Autodesk Inventor part; units mm, degrees
(part 2 of 2)
sketch "Sketch120" plane through (0, 0, 52) normal (0, 0, -1) x (-1, 0, 0)
  line L0 (-5.5, 48.7965) -> (-5.5, 49.7965) projected
  line L1 (-5.5, 47.9965) -> (-5.5, 48.7965) projected
  line L2 (-5.5, 47.9965) -> (-5.5, 45.9965) projected
  line L3 (-5.5, 45.9965) -> (-5.5, 19.7965) projected
  line L4 (-5.5, 19.7965) -> (-5.5, 45.9965) projected
  line L5 (-5.5, 45.9965) -> (-5.5, 47.9965) projected
  line L6 (-5.5, 48.7965) -> (-5.5, 47.9965) projected
  line L7 (-5.5, 49.7965) -> (-5.5, 48.7965) projected
  line L8 (-5.5, -48.7965) -> (-5.5, -49.7965) projected
  line L9 (-5.5, -47.9965) -> (-5.5, -48.7965) projected
  line L10 (-5.5, -47.9965) -> (-5.5, -45.9965) projected
  line L11 (-5.5, -45.9965) -> (-5.5, -19.7965) projected
  line L12 (-5.5, -19.7965) -> (-5.5, -45.9965) projected
  line L13 (-5.5, -45.9965) -> (-5.5, -47.9965) projected
  line L14 (-5.5, -48.7965) -> (-5.5, -47.9965) projected
  line L15 (-5.5, -49.7965) -> (-5.5, -48.7965) projected
  line L16 (-6, 5.3855) -> (-6, 46.7965) projected
  line L17 (-6, -46.7965) -> (-6, -5.3855) projected
  line L18 (-6, 46.7965) -> (-3.5, 46.7965)
  line L19 (-3.5, 46.7965) -> (-3.5, 17.7965)
  line L20 (-3.5, 17.7965) -> (-6, 17.7965)
  line L21 (-6, 17.7965) -> (-6, 46.7965)
  line L22 (-6, -46.7965) -> (-3.5, -46.7965)
  line L23 (-3.5, -46.7965) -> (-3.5, -17.7965)
  line L24 (-3.5, -17.7965) -> (-6, -17.7965)
  line L25 (-6, -17.7965) -> (-6, -46.7965)
  point P0 (0, 0)
  dimension "d491" = 2
  dimension "d492" = 2
  dimension "d493" = 2
  constraints: 16 end point, 4 parallel, 2 horizontal, 2 perpendicular, 1 vertical alignment
  measures "d491" distance between parallel lines of L19 L3
  measures "d492" distance from line of L20 L3.end
  measures "d493" distance from line of L24 L11.end
extrude "Extrusion103" add sketch "Sketch120" along normal blind 2
sketch "Sketch123" plane through (9, -49.7965, 50) normal (1, 0, 0) x (0, 0, -1)
  line L0 (-2, 99.5929) -> (-5, 99.5929)
  line L1 (-5, 99.5929) -> (-5, 69.5929)
  line L2 (-5, 69.5929) -> (-2, 69.5929)
  line L3 (-2, 69.5929) -> (-2, 99.5929)
  line L4 (-3, 69.5929) -> (-32, 69.5929) projected
  line L5 (-3, 98.5929) -> (-3, 97.7929) projected
  line L6 (-3, 69.5929) -> (-35, 69.5929) projected
  line L7 (-19, 69.5929) -> (-19, 30)
  line L8 (-35, 30) -> (-3, 30) projected
  line L9 (0, 49.7965) -> (-70, 49.7965) projected
  line L10 (-2, 0) -> (-5, 0)
  line L11 (-5, 0) -> (-5, 30)
  line L12 (-5, 30) -> (-2, 30)
  line L13 (-2, 30) -> (-2, 0)
  line L14 (-36, 99.5929) -> (-33, 99.5929)
  line L15 (-33, 99.5929) -> (-33, 69.5929)
  line L16 (-33, 69.5929) -> (-36, 69.5929)
  line L17 (-36, 69.5929) -> (-36, 99.5929)
  line L18 (-33, 0) -> (-33, 30)
  line L19 (-36, 30) -> (-36, 0)
  line L20 (-33, 30) -> (-36, 30)
  line L21 (-36, 0) -> (-33, 0)
  point P0 (50, 49.7965)
  dimension "d494" = 2
  constraints: 34 end point, 12 symmetric about line, 2 midpoint, 2 parallel, 1 horizontal, 1 perpendicular, 1 point on line
  measures "d494" distance between parallel lines of L1 L5
extrude "Extrusion105" add sketch "Sketch123" against normal blind 1
sketch "Sketch125" plane through (5.5, -49.7965, 50) normal (1, 0, 0) x (0, 0, -1)
  line L0 (-36, 99.5929) -> (-2, 99.5929) projected
  line L1 (-35, 98.5929) -> (-36, 99.5929) projected
  line L2 (-35, 97.7929) -> (-35, 98.5929) projected
  line L3 (-35, 97.7929) -> (-35.6, 97.7929) projected
  line L4 (-35.6, 97.7929) -> (-35.6, 95.7929) projected
  line L5 (-35.6, 95.7929) -> (-35, 69.5929) projected
  line L6 (-3, 69.5929) -> (-35, 69.5929) projected
  line L7 (-3, 69.5929) -> (-2.4, 95.7929) projected
  line L8 (-2.4, 95.7929) -> (-2.4, 97.7929) projected
  line L9 (-2.4, 97.7929) -> (-3, 97.7929) projected
  line L10 (-3, 98.5929) -> (-3, 97.7929) projected
  line L11 (-2, 99.5929) -> (-3, 98.5929) projected
  line L12 (-2, 0) -> (-36, 0) projected
  line L13 (-3, 1) -> (-2, 0) projected
  line L14 (-3, 1.8) -> (-3, 1) projected
  line L15 (-3, 1.8) -> (-2.4, 1.8) projected
  line L16 (-2.4, 1.8) -> (-2.4, 3.8) projected
  line L17 (-2.4, 3.8) -> (-3, 30) projected
  line L18 (-35, 30) -> (-3, 30) projected
  line L19 (-35, 30) -> (-35.6, 3.8) projected
  line L20 (-35.6, 3.8) -> (-35.6, 1.8) projected
  line L21 (-35.6, 1.8) -> (-35, 1.8) projected
  line L22 (-35, 1) -> (-35, 1.8) projected
  line L23 (-36, 0) -> (-35, 1) projected
  point P0 (50, 49.7965)
extrude "Extrusion106" cut sketch "Sketch125" against normal blind 1
sketch "Sketch126" plane through (0, 0, 52) normal (0, 0, -1) x (-1, 0, 0)
  line L0 (21, 25.6491) -> (10, 19.2983)
  line L1 (10, 19.2983) -> (-1, 25.6491)
  line L2 (-1, 25.6491) -> (-1, 38.3509)
  line L3 (-1, 38.3509) -> (10, 44.7017)
  line L4 (10, 44.7017) -> (21, 38.3509)
  line L5 (21, 38.3509) -> (21, 25.6491)
  line L6 (0, 0) -> (77.78, 0) construction
  line L7 (21, -25.6491) -> (10, -19.2983)
  line L8 (10, -19.2983) -> (-1, -25.6491)
  line L9 (-1, -25.6491) -> (-1, -38.3509)
  line L10 (-1, -38.3509) -> (10, -44.7017)
  line L11 (10, -44.7017) -> (21, -38.3509)
  line L12 (21, -38.3509) -> (21, -25.6491)
  point P0 (10, 32)
  dimension "d499" = 32
  dimension "d500" = 22
  dimension "d501" = 10
  constraints: 26 end point, 6 symmetric about line, 1 horizontal, 1 vertical, 13 other
  measures "d499" vertical distance of L6.start point (10, 32)
  measures "d500" distance between parallel lines of L2 L5
  measures "d501" horizontal distance of L6.start point (10, 32)
extrude "Extrusion107" cut sketch "Sketch126" against normal through all
sketch "Sketch128" plane through (4.5, -49.7965, 50) normal (1, 0, 0) x (0, 0, -1)
  line L0 (-36, 99.5929) -> (-2, 99.5929) construction
  line L1 (-35, 98.5929) -> (-36, 99.5929) projected
  line L2 (-35, 97.7929) -> (-35, 98.5929) projected
  line L3 (-35.6, 97.7929) -> (-35, 97.7929) projected
  line L4 (-35.6, 95.7929) -> (-35.6, 97.7929) projected
  line L5 (-35, 69.5929) -> (-35.6, 95.7929) projected
  line L6 (-3, 69.5929) -> (-35, 69.5929) projected
  line L7 (-2.4, 95.7929) -> (-3, 69.5929) projected
  line L8 (-2.4, 97.7929) -> (-2.4, 95.7929) projected
  line L9 (-3, 97.7929) -> (-2.4, 97.7929) projected
  line L10 (-3, 98.5929) -> (-3, 97.7929) projected
  line L11 (-2, 99.5929) -> (-3, 98.5929) projected
  line L12 (-2.4, 97.7929) -> (-2.4, 99.1929)
  line L13 (-2.4, 99.1929) -> (-3, 98.5929)
  line L14 (-3, 98.5929) -> (-3, 97.7929)
  line L15 (-2.4, 97.7929) -> (-3, 97.7929)
  line L16 (-35.6, 97.7929) -> (-35.6, 99.1929)
  line L17 (-35.6, 99.1929) -> (-35, 98.5929)
  line L18 (-35, 97.7929) -> (-35, 98.5929)
  line L19 (-35, 97.7929) -> (-35.6, 97.7929)
  point P0 (50, 49.7965)
  constraints: 16 end point, 5 collinear, 2 point on line, 1 parallel, 1 perpendicular, 1 vertical
extrude "Extrusion108" cut sketch "Sketch128" along normal blind 3.5
sketch "Sketch129" plane through (4.5, -49.7965, 50) normal (1, 0, 0) x (0, 0, -1)
  line L0 (-36, 99.5929) -> (-2, 99.5929) projected
  line L1 (-35.6, 99.1929) -> (-36, 99.5929) projected
  line L2 (-35.6, 99.1929) -> (-35.6, 95.7929) projected
  line L3 (-35, 69.5929) -> (-35.6, 95.7929) projected
  line L4 (-3, 69.5929) -> (-35, 69.5929) construction
  line L5 (-2.4, 95.7929) -> (-3, 69.5929) projected
  line L6 (-2.4, 99.1929) -> (-2.4, 95.7929) projected
  line L7 (-2, 99.5929) -> (-2.4, 99.1929) projected
  line L8 (-35, 69.5929) -> (-35, 99.5929)
  line L9 (-35, 99.5929) -> (-3, 99.5929)
  line L10 (-3, 99.5929) -> (-3, 69.5929)
  line L11 (-35, 99.5929) -> (-34, 99.5929)
  line L12 (-34, 99.5929) -> (-34, 97.5929)
  line L13 (-34, 97.5929) -> (-35, 97.5929)
  line L14 (-35, 97.5929) -> (-35, 99.5929)
  line L15 (-35, 99.5929) -> (-36, 99.5929)
  line L16 (-35, 97.5929) -> (-36, 97.5929)
  line L17 (-36, 97.5929) -> (-36, 99.5929)
  point P0 (50, 49.7965)
  dimension "d506" = 1
  dimension "d507" = 28
  dimension "d508" = 2
  constraints: 20 end point, 4 parallel, 4 perpendicular, 3 point on line, 2 horizontal
  measures "d506" distance of L12.end L13.end
  measures "d507" distance between parallel lines of L4 L13
  measures "d508" distance of L11.end L12.end
extrude "Extrusion109" add sketch "Sketch129" along normal blind 3.5 contours L0 L8 L16 L2 L1 | L1 L2 L16 L17 | L0 L12 L13 L8
mirror "Mirror1" about plane through (0, 0, 0) normal (0, 1, 0) of "Extrusion108", "Extrusion109"
chamfer "Chamfer4" distance 1 angle 45 2 edges at (6.25, -49.7965, 84) (6.25, 49.7965, 84)
sketch "Sketch131" plane through (0, 0, 82) normal (0, 0, -1) x (-1, 0, 0)
  circle A0 centre (-30, 0) radius 16.5 projected
  line L0 (-27.0179, 46.7965) -> (-9, 46.7965) projected
  line L1 (-54.0359, 0) -> (-27.0179, 46.7965) projected
  line L2 (-27.0179, -46.7965) -> (-54.0359, 0) projected
  line L3 (-9, -46.7965) -> (-27.0179, -46.7965) projected
  line L4 (-9, -19.7965) -> (-9, -46.7965) projected
  line L5 (-9, 19.7965) -> (-9, -19.7965) projected
  line L6 (-9, 46.7965) -> (-9, 19.7965) projected
  point P0 (0, 0)
extrude "Extrusion111" add sketch "Sketch131" along normal blind 2
sketch "Sketch132" plane through (0, 0, 52) normal (0, 0, -1) x (-1, 0, 0)
  line L0 (21, 38.3509) -> (21, 25.6491) projected
  line L1 (21, 25.6491) -> (10, 19.2983) projected
  line L2 (10, 19.2983) -> (-1, 25.6491) projected
  line L3 (-1, 25.6491) -> (-1, 38.3509) projected
  line L4 (-1, 38.3509) -> (10, 44.7017) projected
  line L5 (10, 44.7017) -> (21, 38.3509) projected
  line L6 (21, -25.6491) -> (21, -38.3509) projected
  line L7 (21, -38.3509) -> (10, -44.7017) projected
  line L8 (10, -44.7017) -> (-1, -38.3509) projected
  line L9 (-1, -38.3509) -> (-1, -25.6491) projected
  line L10 (-1, -25.6491) -> (10, -19.2983) projected
  line L11 (10, -19.2983) -> (21, -25.6491) projected
  arc A0 (38.8444, 24.1666) -> (21.1556, 24.1666) centre (30, 19.5) ccw projected
  line L12 (45, 12.5) -> (38.8444, 24.1666) projected
  line L13 (45, -12.5) -> (45, 12.5) projected
  line L14 (38.5, -12.5) -> (45, -12.5) projected
  line L15 (38.5, -19.5) -> (38.5, -12.5) projected
  line L16 (21.5, -19.5) -> (38.5, -19.5) projected
  line L17 (21.5, -12.5) -> (21.5, -19.5) projected
  line L18 (15, -12.5) -> (21.5, -12.5) projected
  line L19 (15, 12.5) -> (15, -12.5) projected
  line L20 (21.1556, 24.1666) -> (15, 12.5) projected
  line L21 (-3.5, 46.7965) -> (-3.5, 17.7965) projected
  line L22 (-3.5, 17.7965) -> (-6, 17.7965) projected
  line L23 (-6, 17.7965) -> (-6, 5.3855) projected
  arc A1 (-6, -5.3855) -> (-6, 5.3855) centre (0, 0) ccw projected
  line L24 (-6, -17.7965) -> (-6, -5.3855) projected
  line L25 (-6, -17.7965) -> (-3.5, -17.7965) projected
  line L26 (-3.5, -17.7965) -> (-3.5, -46.7965) projected
  line L27 (-3.5, -46.7965) -> (27.0179, -46.7965) projected
  line L28 (27.0179, -46.7965) -> (54.0359, 0) projected
  line L29 (27.0179, 46.7965) -> (54.0359, 0) projected
  line L30 (27.0179, 46.7965) -> (-3.5, 46.7965) projected
extrude "Extrusion112" add sketch "Sketch132" along normal blind 2
sketch "Sketch134" plane through (0, 0, 50) normal (0, 0, -1) x (-1, 0, 0)
  line L0 (21, 38.3509) -> (21, 25.6491) projected
  line L1 (21, 25.6491) -> (10, 19.2983) projected
  line L2 (21, 25.6491) -> (10, 19.2983) projected
  line L3 (10, 19.2983) -> (-1, 25.6491) projected
  line L4 (-1, 25.6491) -> (-1, 38.3509) projected
  line L5 (-1, 38.3509) -> (10, 44.7017) projected
  line L6 (10, 44.7017) -> (21, 38.3509) projected
  line L7 (21, 38.3509) -> (21, 25.6491) projected
  line L8 (21, -38.3509) -> (10, -44.7017) projected
  line L9 (10, -44.7017) -> (-1, -38.3509) projected
  line L10 (-1, -38.3509) -> (-1, -25.6491) projected
  line L11 (-1, -25.6491) -> (10, -19.2983) projected
  line L12 (10, -19.2983) -> (21, -25.6491) projected
  line L13 (21, -25.6491) -> (21, -38.3509) projected
  line L14 (38.8444, 24.1666) -> (45, 12.5) projected
  line L15 (45, 12.5) -> (45, -12.5) projected
  line L16 (45, -12.5) -> (38.5, -12.5) projected
  line L17 (38.5, -12.5) -> (38.5, -19.5) projected
  line L18 (38.5, -19.5) -> (21.5, -19.5) projected
  line L19 (21.5, -19.5) -> (21.5, -12.5) projected
  line L20 (21.5, -12.5) -> (15, -12.5) projected
  line L21 (15, -12.5) -> (15, 12.5) projected
  line L22 (15, 12.5) -> (21.1556, 24.1666) projected
  arc A0 (38.8444, 24.1666) -> (21.1556, 24.1666) centre (30, 19.5) ccw projected
  circle A1 centre (0, 0) radius 8.0625 projected
  line L23 (28.75, -49.7965) -> (57.5, 0) projected
  line L24 (28.75, 49.7965) -> (57.5, 0) projected
  line L25 (28.75, 49.7965) -> (-9, 49.7965) projected
  line L26 (-9, 49.7965) -> (-9, -49.7965) projected
  line L27 (-9, -49.7965) -> (28.75, -49.7965) projected
extrude "Extrusion113" add sketch "Sketch134" against normal blind 70 contours L0 L1 L3 L4 L5 L6 | L8 L9 L10 L11 L12 L13
sketch "Sketch135" plane through (0, 0, 50) normal (0, 0, -1) x (-1, 0, 0)
  circle A0 centre (0, 0) radius 42.5 construction
  circle A1 centre (26.2333, -33.4374) radius 3.5 construction
  circle A2 centre (15.841, -39.4374) radius 3.5 construction
  circle A3 centre (-17.8508, -38.5694) radius 3.5 construction
  circle A4 centre (-30.1381, -29.9658) radius 3.5 construction
  line L0 (26.2333, -33.4374) -> (15.841, -39.4374)
  line L1 (-17.8508, -38.5694) -> (-30.1381, -29.9658)
  line L2 (0, 0) -> (21.0372, -36.4374) construction
  line L3 (21.0372, -36.4374) -> (-23.9944, -34.2676) construction
  line L4 (0, 0) -> (-23.9944, -34.2676) construction
  line L5 (0, 0) -> (16.8866, 0) construction
  circle A5 centre (26.2333, 33.4374) radius 3.5 construction
  circle A6 centre (15.841, 39.4374) radius 3.5 construction
  circle A7 centre (-17.8508, 38.5694) radius 3.5 construction
  circle A8 centre (-30.1381, 29.9658) radius 3.5 construction
  circle A9 centre (0, 0) radius 39 construction
  circle A10 centre (0, 0) radius 46 construction
  arc A11 (30.8761, -34.0979) -> (26.1775, -28.9091) centre (28.5268, -31.5035) ccw
  arc A12 (11.9473, -37.125) -> (14.0917, -43.7884) centre (13.0195, -40.4567) ccw
  arc A13 (14.0917, -43.7884) -> (30.8761, -34.0979) centre (0, 0) ccw
  arc A14 (11.9473, -37.125) -> (26.1775, -28.9091) centre (0, 0) ccw
  line L6 (23, -39.8372) -> (19.5, -33.775)
  arc A15 (-16.3278, -43.0047) -> (-13.8431, -36.4605) centre (-15.0855, -39.7326) ccw
  arc A16 (-29.527, -25.4785) -> (-34.8268, -30.0516) centre (-32.1769, -27.765) ccw
  arc A17 (-29.527, -25.4785) -> (-13.8431, -36.4605) centre (0, 0) ccw
  arc A18 (-34.8268, -30.0516) -> (-16.3278, -43.0047) centre (0, 0) ccw
  circle A19 centre (26.2333, 33.4374) radius 3.5 construction
  line L7 (26.2333, 33.4374) -> (15.841, 39.4374)
  circle A20 centre (15.841, 39.4374) radius 3.5 construction
  line L8 (21.0372, 36.4374) -> (-23.9944, 34.2676) construction
  circle A21 centre (-17.8508, 38.5694) radius 3.5 construction
  circle A22 centre (-30.1381, 29.9658) radius 3.5 construction
  line L9 (-17.8508, 38.5694) -> (-30.1381, 29.9658)
  arc A23 (26.1775, 28.9091) -> (30.8761, 34.0979) centre (28.5268, 31.5035) ccw
  arc A24 (14.0917, 43.7884) -> (11.9473, 37.125) centre (13.0195, 40.4567) ccw
  arc A25 (30.8761, 34.0979) -> (14.0917, 43.7884) centre (0, 0) ccw
  arc A26 (26.1775, 28.9091) -> (11.9473, 37.125) centre (0, 0) ccw
  line L10 (23, 39.8372) -> (19.5, 33.775)
  arc A27 (-13.8431, 36.4605) -> (-16.3278, 43.0047) centre (-15.0855, 39.7326) ccw
  arc A28 (-34.8268, 30.0516) -> (-29.527, 25.4785) centre (-32.1769, 27.765) ccw
  arc A29 (-13.8431, 36.4605) -> (-29.527, 25.4785) centre (0, 0) ccw
  arc A30 (-16.3278, 43.0047) -> (-34.8268, 30.0516) centre (0, 0) ccw
  dimension "d549" = 85
  dimension "d550" = 7
  dimension "d551" = 7
  dimension "d552" = 7
  dimension "d553" = 7
  dimension "d554" = 12
  dimension "d555" = 60
  dimension "d556" = 65
  dimension "d557" = 15
  dimension "d558" = 3
  dimension "d560" = 3
  dimension "d561" = 3
  constraints: 46 point on circle, 31 centre point, 24 symmetric about line, 22 end point, 10 tangent, 4 coincident, 4 concentric, 2 midpoint, 2 point on line, 1 horizontal, 1 perpendicular, 16 other
  measures "d549" diameter of A0
  measures "d550" diameter of A1
  measures "d551" diameter of A2
  measures "d552" diameter of A3
  measures "d553" diameter of A4
  measures "d554" distance of L0.start L0.end
  measures "d555" angle of L2 L5
  measures "d556" angle of L2 L4
  measures "d557" distance of L1.start L1.end
  measures "d558" distance of L0.start A11.centre
  measures "d560" distance of L1.start A15.centre
  measures "d561" distance of L1.end A16.centre
extrude "Extrusion114" cut sketch "Sketch135" against normal blind 3 contours A13 L6 A14 A11 | A13 A12 A14 L6 | A26 L10 A25 A23 | A26 A24 A25 L10
extrude "Extrusion115" cut sketch "Sketch135" against normal blind 33 contours A18 A16 A17 A15 | A29 A28 A30 A27
body "Solid2"
